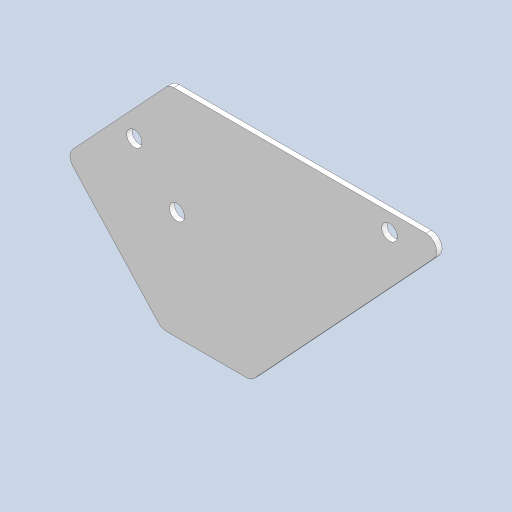
# Autodesk Inventor part: meow
Saved by Autodesk Inventor 2024.2 (Build 282272000, 272)
## iProperties
Created: 2024-01-05
Part Number: meow
Material: Acetal Resin, White
Document SubType Name: Modeling
Designer: reima
Density: 1.425 g/cm^3
Appearance: Smooth - White
Author: reima
Autodesk Inventor part; units mm, degrees
ref_plane "YZ Plane" through (0, 0, 0) normal (1, 0, 0) x (0, 1, 0)
ref_plane "XZ Plane" through (0, 0, 0) normal (0, 1, 0) x (-1, 0, 0)
ref_plane "Work Plane1" through (456.7, 53.6703, -0.1016) normal (0, 0, 1) x (0, 1, 0)
sketch "Sketch1" plane through (456.7, 53.6703, -0.1016) normal (0, 0, 1) x (0, 1, 0)
  circle A0 centre (-38.1, 19.05) radius 2.3114 construction
  circle A1 centre (-38.1, 31.75) radius 2.3114 construction
  circle A2 centre (-38.1, 31.75) radius 47.625 construction
  line L0 (-85.725, 31.75) -> (-85.725, -73.025) construction
  line L1 (-85.725, -73.025) -> (-69.85, -73.025) construction
  circle A3 centre (-39.624, -73.025) radius 30.226 construction
  line L2 (-63.4579, -9.6878) -> (-11.6843, -57.7145)
  line L3 (-6.35, -55.3867) -> (-6.35, 19.9759)
  line L4 (-70.4888, 2.6423) -> (-70.4888, 9.8614)
  arc A4 (-11.6843, -57.7145) -> (-6.35, -55.3867) centre (-9.525, -55.3867) ccw
  line L5 (-63.4579, -9.6878) -> (-69.473, -4.1079)
  line L6 (-70.4888, 2.6423) -> (-70.4888, -1.7802)
  arc A5 (-70.4888, -1.7802) -> (-69.473, -4.1079) centre (-67.3138, -1.7802) ccw
  circle A6 centre (-25.4, 31.75) radius 2.3114 projected
  line L7 (-70.4888, -1.7802) -> (-70.4888, 22.2286)
  line L8 (-7.3657, 22.3036) -> (-37.3903, 50.1552)
  arc A7 (-6.35, 19.9759) -> (-7.3657, 22.3036) centre (-9.525, 19.9759) ccw
  line L9 (-69.466, 24.5628) -> (-41.7017, 50.1618)
  arc A8 (-37.3903, 50.1552) -> (-41.7017, 50.1618) centre (-39.5495, 47.8275) ccw
  arc A9 (-69.466, 24.5628) -> (-70.4888, 22.2286) centre (-67.3138, 22.2286) ccw
  circle A10 centre (-38.1, 19.05) radius 2.3114 projected
  circle A11 centre (-25.4, 19.05) radius 2.3114 projected
  circle A12 centre (-11.5316, -44.45) radius 2.3368
  circle A13 centre (-11.5316, -44.45) radius 2.1844 construction
  point P0 (-53.6703, 456.7)
  point P1 (-70.4888, -3.1657)
  point P2 (6.35, -48.768)
  point P3 (-6.35, 21.3614)
  point P4 (-19.05, 12.7)
  point P5 (-70.4888, 23.6198)
  dimension "d0" = 95.25
  dimension "d1" = 104.775
  dimension "d2" = 15.875
  dimension "d3" = 60.452
  dimension "d4" = 0
  dimension "d5" = 30.226
  dimension "d8" = 3.175
  dimension "d16" = 3.175
  dimension "d19" = 12.7
  dimension "d20" = 25.4
  dimension "d22" = 3.175
  dimension "d23" = 4.6736
  dimension "d26" = 63.5
  dimension "d29" = 0
  constraints: 20 end point, 14 tangent, 12 point on circle, 9 point on line, 8 centre point, 3 vertical, 1 coincident, 1 equal radius, 1 parallel, 1 perpendicular, 2 other
  measures "d0" diameter of A2
  measures "d1" distance of L0.start L0.end
  measures "d2" distance of L0.end L1.end
  measures "d3" diameter of A3
  measures "d4" vertical distance of L0.end A3.centre
  measures "d5" distance of L1.end A3.centre
  measures "d8" radius of A4
  measures "d16" radius of A5
  measures "d19" distance from line of point (-19.05, 12.7) L3
  measures "d20" distance of L6.end point (-70.489, 23.62)
  measures "d22" radius of A8
  measures "d23" diameter of A12
  measures "d26" vertical distance of A11.centre A12.centre
  measures "d29" distance of A12.centre A13.centre
extrude "Extrusion2" add sketch "Sketch1" along normal blind 1.5875 contours L5 A5 L6 L4 L7 A9 L9 A8 L8 A7 L3 A4 L2 | A11
body "Solid2"
